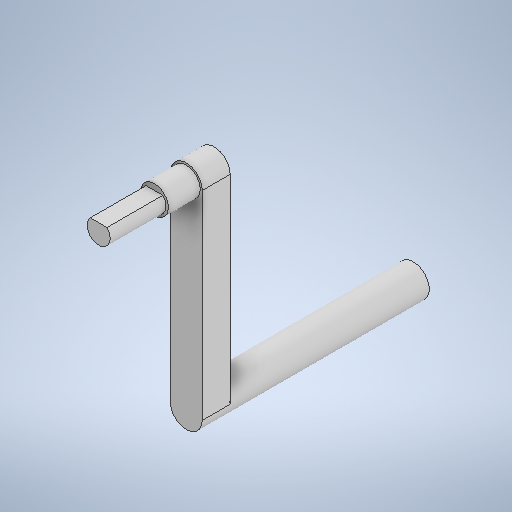
# Autodesk Inventor part: HandCrank
Saved by Autodesk Inventor 2025.1 (Build 291241000, 241)
## iProperties
Created: 2025-02-27
Part Number: HandCrank
Material: Generic
Document SubType Name: Modeling
Designer: frede
Density: 1 g/cm^3
Appearance: Default
Description: Bliver lavet om til motor
Author: frede
Autodesk Inventor part; units mm, degrees
ref_plane "YZ Plane" through (0, 0, 0) normal (1, 0, 0) x (0, 1, 0)
ref_plane "XZ Plane" through (0, 0, 0) normal (0, 1, 0) x (-1, 0, 0)
ref_plane "XY Plane" through (0, 0, 0) normal (0, 0, 1) x (1, 0, 0)
sketch "Sketch1" plane through (0, 0, 0) normal (1, 0, 0) x (0, 1, 0)
  line L0 (0, 0) -> (2.9, 0)
  line L1 (2.9, 0) -> (2.9, -14)
  line L2 (0, -14) -> (0, 0)
  line L3 (2.9, -14) -> (3.5, -14)
  line L4 (3.5, -14) -> (3.5, -22)
  line L5 (3.5, -22) -> (0, -22)
  line L6 (0, -22) -> (0, -14)
  dimension "d0" = 14
  dimension "d1" = 3.5
  dimension "d2" = 8
  dimension "d3" = 2.9
  constraints: 14 end point, 3 parallel, 2 horizontal, 2 perpendicular
  measures "d0" distance of L1.end L0.end
  measures "d1" distance of L4.end L5.end
  measures "d2" distance of L3.end L4.end
  measures "d3" distance between parallel lines of L2 L1
revolve "Revolution1" add sketch "Sketch1" angle 360 about axis through (0, 0, -22) along (0, 0, 1)
sketch "Sketch2" plane through (0, 0, -22) normal (0, 0, -1) x (-1, 0, 0)
  circle A0 centre (0, 0) radius 4
  line L0 (-4, 0) -> (4, 0)
  line L1 (4, 0) -> (4, -50)
  line L2 (4, -50) -> (-4, -50)
  line L3 (-4, -50) -> (-4, 0)
  circle A1 centre (0, -50) radius 4
  point P0 (4, 0)
  dimension "d5" = 8
  dimension "d6" = 50
  constraints: 8 end point, 2 parallel, 1 coincident, 1 horizontal, 1 midpoint, 1 perpendicular, 6 other
  measures "d6" distance of L0.end L1.end
extrude "Extrusion1" add sketch "Sketch2" along normal blind 7
sketch "Sketch3" plane through (0, 0, -29) normal (0, 0, -1) x (-1, 0, 0)
  arc A0 (-4, -50) -> (4, -50) centre (0, -50) ccw projected
  circle A1 centre (0, -50) radius 4
  point P0 (0, 0)
  point P1 (4, -50)
  point P2 (-4, -50)
  constraints: 1 centre point, 1 coincident
extrude "Extrusion2" add sketch "Sketch3" along normal blind 50
sketch "Sketch4" plane through (0, 0, 0) normal (0, 0, 1) x (1, 0, 0)
  line L0 (2.1, 2) -> (-2.1, 2)
  arc A0 (2.1, 2) -> (-2.1, 2) centre (0, 0) ccw
  dimension "d11" = 2
  constraints: 2 end point, 2 point on circle, 1 centre point, 1 coincident, 1 horizontal
  measures "d11" distance from line of point (0, 0) L0
extrude "Extrusion3" cut sketch "Sketch4" against normal up to surface (14 mm away)
body "Solid1"
